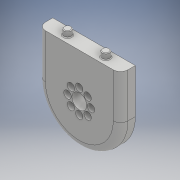
# Autodesk Inventor part: arm_segment_3_2b
Saved by Autodesk Inventor 2018 (Build 220112000, 112)
## iProperties
Created: 2018-04-12
Part Number: arm_segment_3_2b
Material: Generic
Document SubType Name: Modeling
Designer: mshaw2
Density: 1 g/cm^3
Appearance: Default
Author: mshaw2
## iProperties of the stored document arm_segment_3_2b_3DPrint.ipt
Created: 2018-04-15
Part Number: arm_segment_3_2b_3DPrint
Material: Generic
Document SubType Name: Modeling
Designer: mshaw2
Density: 1 g/cm^3
Appearance: Default
Author: mshaw2
Autodesk Inventor part; units mm, degrees
ref_plane "YZ Plane" through (0, 0, 0) normal (1, 0, 0) x (0, 1, 0)
ref_plane "XZ Plane" through (0, 0, 0) normal (0, 1, 0) x (-1, 0, 0)
ref_plane "XY Plane" through (0, 0, 0) normal (0, 0, 1) x (1, 0, 0)
sketch "Sketch1" plane through (0, 0, 0) normal (0, 1, 0) x (-1, 0, 0)
  circle A0 centre (0, 0) radius 11.5 construction
  circle A1 centre (0, 0) radius 4 construction
  circle A2 centre (0, 0) radius 5
  circle A3 centre (0, 0) radius 8 construction
  circle A4 centre (8, 0) radius 1.45
  circle A5 centre (5.6569, 5.6569) radius 1.45
  circle A6 centre (0, 8) radius 1.45
  circle A7 centre (-5.6569, 5.6569) radius 1.45
  circle A8 centre (-8, 0) radius 1.45
  circle A9 centre (-5.6569, -5.6569) radius 1.45
  circle A10 centre (0, -8) radius 1.45
  circle A11 centre (5.6569, -5.6569) radius 1.45
  arc A12 (-28, 0) -> (28, 0) centre (0, 0) ccw
  line L0 (28, 0) -> (28, 34)
  line L1 (28, 0) -> (62, 0) construction
  line L2 (28, 34) -> (-28, 34)
  line L3 (-28, 34) -> (-28, 0)
  dimension "d4" = 16
  dimension "d2" = 1
  dimension "d3" = 10
  dimension "d5" = 2.9
  dimension "d6" = 360
  dimension "d7" = 28
  dimension "d8" = 34
  dimension "d9" = 90
  constraints: 12 centre point, 8 end point, 2 coincident, 2 perpendicular, 2 point on circle, 2 tangent, 1 horizontal, 1 horizontal alignment, 1 parallel, 1 vertical, 23 other
  measures "d2" radial gap between concentric circles of A1 A2
  measures "d3" diameter of A2
  measures "d5" diameter of A4
  measures "d7" radius of A12
  measures "d8" distance of L0.start L0.end
  measures "d9" angle of L1 L0
extrude "Extrusion1" add sketch "Sketch1" along normal blind 10
sketch "Sketch2" plane through (0, 10, 0) normal (0, 1, 0) x (1, 0, 0)
  circle A0 centre (0, 0) radius 11.5 projected
  circle A1 centre (-5.6569, -5.6569) radius 1.45 projected
  circle A2 centre (-8, 0) radius 1.45 projected
  circle A3 centre (-5.6569, 5.6569) radius 1.45 projected
  circle A4 centre (0, 8) radius 1.45 projected
  circle A5 centre (5.6569, 5.6569) radius 1.45 projected
  circle A6 centre (0, 0) radius 5 projected
  circle A7 centre (8, 0) radius 1.45 projected
  circle A8 centre (5.6569, -5.6569) radius 1.45 projected
  circle A9 centre (5.6569, -5.6569) radius 1.45 projected
  circle A10 centre (0, -8) radius 1.45 projected
extrude "Extrusion2" add sketch "Sketch2" along normal blind 4.5
sketch "Sketch3" plane through (0, 0, 0) normal (0, -1, 0) x (1, 0, 0)
  circle A0 centre (8, 0) radius 1.45 construction
  circle A1 centre (5.6569, -5.6569) radius 1.45 construction
  circle A2 centre (0, -8) radius 1.45 construction
  circle A3 centre (-5.6569, -5.6569) radius 1.45 construction
  circle A4 centre (-8, 0) radius 1.45 construction
  circle A5 centre (0, 0) radius 5 construction
  circle A6 centre (-5.6569, -5.6569) radius 1.45 construction
  circle A7 centre (0, -8) radius 1.45 construction
  circle A8 centre (5.6569, -5.6569) radius 1.45 construction
  circle A9 centre (8, 0) radius 1.45 construction
  circle A10 centre (5.6569, 5.6569) radius 1.45 construction
  circle A11 centre (0, 8) radius 1.45 construction
  circle A12 centre (-5.6569, 5.6569) radius 1.45 construction
  circle A13 centre (-8, 0) radius 1.45 construction
  arc A14 (-28, 0) -> (28, 0) centre (0, 0) ccw construction
  line L0 (28, 34) -> (28, 0) construction
  line L1 (-28, 34) -> (28, 34) construction
  line L2 (-28, 0) -> (-28, 34) construction
hole "Hole1" at (5.6569, 0, 5.6569) at (8, 0, 0) at (5.6569, 0, -5.6569) at (0, 0, -8) at (-5.6569, 0, -5.6569) at (-8, 0, 0) at (-5.6569, 0, 5.6569) at (0, 0, 8) direction (0, 1, 0) diameter 5 depth 10.5
sketch "Sketch4" plane through (0, 10, 0) normal (0, 1, 0) x (1, 0, 0)
  line L0 (28, -34) -> (28, 0) projected
  line L1 (-28, 0) -> (-28, -34) projected
  line L2 (28, -34) -> (-28, -34)
  line L3 (-28, -34) -> (-28, -30)
  line L4 (-28, -30) -> (28, -30)
  line L5 (28, -30) -> (28, -34)
  point P0 (0, 0)
  dimension "d21" = 4
  constraints: 8 end point, 2 parallel, 1 horizontal, 1 perpendicular, 1 point on line
  measures "d21" distance of L2.end L3.end
extrude "Extrusion6" cut sketch "Sketch4" against normal through all
sketch "Sketch9" plane through (-28, 10, 30) normal (0, 0, 1) x (1, 0, 0)
  line L0 (56, -62) -> (56, 0)
  line L1 (0, 0) -> (56, 0)
  line L2 (56, 0) -> (56, -10)
  line L3 (56, -10) -> (0, -10)
  line L4 (0, -10) -> (0, 0)
  line L5 (0, -62) -> (0, 0) construction
  line L6 (0, -5) -> (56, -5) construction
  circle A0 centre (15, -5) radius 2.5
  circle A1 centre (41, -5) radius 2.5
  point P0 (28, -10)
  point P1 (28, -72)
  dimension "d64" = 10
  dimension "d65" = 15
  dimension "d66" = 15
  dimension "d67" = 5
  dimension "d68" = 5
  constraints: 14 end point, 4 point on line, 2 centre point, 2 coincident, 2 parallel, 1 horizontal, 1 midpoint, 1 perpendicular
  measures "d64" distance of L1.end L2.end
  measures "d65" distance from line of L0 point (41, -5)
  measures "d66" distance from line of point (15, -5) L4
  measures "d67" diameter of A0
  measures "d68" diameter of A1
extrude "Extrusion7" add sketch "Sketch9" along normal blind 4 contours A0 | A1
fillet "Fillet4" radius 0.5 4 edges at (-15.5, 5, 30) (-15.5, 5, 34) (10.5, 5, 34) (10.5, 5, 30)
fillet "Fillet5" radius 5 4 edges at (-28, 0, 15) (28, 0, 15) (0, 0, -28) (-11.5, 10, 0)
body "Solid1"
